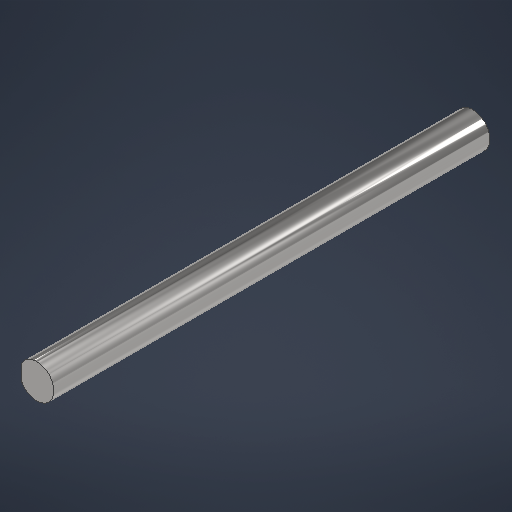
# Autodesk Inventor part: drive_shaft_6mm_d
Saved by Autodesk Inventor 2026 (Build 300175050, 175E)
## iProperties
Created: 2025-06-13
Part Number: drive_shaft_6mm_d
Material: Generic
Document SubType Name: Modeling
Designer: satom
Density: 1 g/cm^3
Appearance: Default
Author: satom
Autodesk Inventor part; units mm, degrees
ref_plane "YZ Plane" through (0, 0, 0) normal (1, 0, 0) x (0, 1, 0)
ref_plane "XZ Plane" through (0, 0, 0) normal (0, 1, 0) x (-1, 0, 0)
ref_plane "XY Plane" through (0, 0, 0) normal (0, 0, 1) x (1, 0, 0)
sketch "Sketch1" plane through (0, 0, 0) normal (0, 0, 1) x (1, 0, 0)
  arc A0 (-2.6, -1.4967) -> (-2.6, 1.4967) centre (0, 0) ccw
  line L0 (-2.6, 1.4967) -> (-2.6, -1.4967)
  line L1 (0, 0) -> (3, 0) construction
  line L2 (3, 3.2672) -> (3, -2.6069) construction
  dimension "d0" = 6
  dimension "d1" = 5.6
  constraints: 6 end point, 3 point on circle, 2 vertical, 1 centre point, 1 coincident, 1 horizontal, 1 perpendicular
  measures "d0" diameter of A0
  measures "d1" distance between parallel lines of L2 L0
extrude "Extrusion1" add sketch "Sketch1" along normal blind 76.2
body "Solid1"
